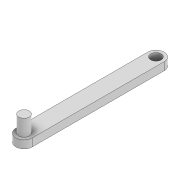
# Autodesk Inventor part: manivela
Saved by Autodesk Inventor 2021 (Build 250183000, 183)
## iProperties
Created: 2021-05-03
Part Number: manivela
Material: Generic
Document SubType Name: Modeling
Designer: Santiago Suárez
Density: 1 g/cm^3
Appearance: Default
Author: Santiago Suárez
Autodesk Inventor part; units mm, degrees
ref_plane "YZ Plane" through (0, 0, 0) normal (1, 0, 0) x (0, 1, 0)
ref_plane "XZ Plane" through (0, 0, 0) normal (0, 1, 0) x (-1, 0, 0)
ref_plane "XY Plane" through (0, 0, 0) normal (0, 0, 1) x (1, 0, 0)
sketch "Sketch1" plane through (0, 0, 0) normal (0, 1, 0) x (-1, 0, 0)
  line L0 (0, 0) -> (0, -200) construction
  arc A0 (12.5, 0) -> (-12.5, 0) centre (0, 0) ccw
  arc A1 (-12.5, -200) -> (12.5, -200) centre (0, -200) ccw
  line L1 (12.5, -200) -> (12.5, 0)
  line L2 (-12.5, -200) -> (-12.5, 0)
  dimension "d0" = 200
  dimension "d3" = 25
  dimension "d4" = 25
  constraints: 6 end point, 4 point on circle, 4 tangent, 2 centre point, 1 vertical
  measures "d0" distance of L0.start L0.end
  measures "d3" diameter of A0
  measures "d4" diameter of A1
extrude "Extrusion1" add sketch "Sketch1" along normal mid plane 12
sketch "Sketch2" plane through (0, 6, 0) normal (0, 1, 0) x (1, 0, 0)
  circle A0 centre (0, 0) radius 8
  dimension "d7" = 16
  constraints: 1 centre point, 1 coincident
  measures "d7" diameter of A0
extrude "Extrusion2" add sketch "Sketch2" along normal blind 25
sketch "Sketch3" plane through (0, 6, 0) normal (0, 1, 0) x (1, 0, 0)
  circle A0 centre (0, 200) radius 8
  point P0 (0, 0)
  dimension "d10" = 16
  constraints: 1 centre point
  measures "d10" diameter of A0
extrude "Extrusion3" cut sketch "Sketch3" against normal blind 12
body "Solid1"
